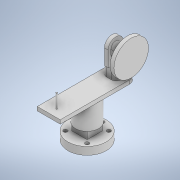
# Autodesk Inventor part: herramienta5
Saved by Autodesk Inventor 2022.3 (Build 263350000, 350)
## iProperties
Created: 2023-06-16
Part Number: herramienta5
Material: Generic
Document SubType Name: Modeling
Designer: crist
Density: 1 g/cm^3
Appearance: Default
Author: crist
Autodesk Inventor part; units mm, degrees
ref_plane "YZ Plane" through (0, 0, 0) normal (1, 0, 0) x (0, 1, 0)
ref_plane "XZ Plane" through (0, 0, 0) normal (0, 1, 0) x (-1, 0, 0)
ref_plane "XY Plane" through (0, 0, 0) normal (0, 0, 1) x (1, 0, 0)
sketch "Sketch1" plane through (0, 0, 0) normal (0, 1, 0) x (-1, 0, 0)
  line L0 (10, 10) -> (-10, 10)
  line L1 (-10, 10) -> (-10, -10)
  line L2 (-10, -10) -> (10, -10)
  line L3 (10, -10) -> (10, 10)
  line L4 (10, 10) -> (-10, -10) construction
  line L5 (-10, 10) -> (10, -10) construction
  point P0 (0, 0)
  dimension "d0" = 20
  dimension "d1" = 20
  constraints: 12 end point, 2 midpoint, 2 parallel, 1 horizontal, 1 perpendicular
  measures "d0" distance of L2.end L1.end
  measures "d1" distance of L1.end L0.end
extrude "Extrusion1" add sketch "Sketch1" along normal blind 20
sketch "Sketch2" plane through (0, 20, 0) normal (0, 1, 0) x (1, 0, 0)
  circle A0 centre (0, 0) radius 15
  dimension "d4" = 30
  constraints: 1 centre point, 1 coincident
  measures "d4" diameter of A0
extrude "Extrusion2" add sketch "Sketch2" along normal blind 30
sketch "Sketch3" plane through (0, 50, 0) normal (0, 1, 0) x (1, 0, 0)
  line L0 (-15, -50) -> (15, -50)
  line L1 (15, -50) -> (15, 50)
  line L2 (15, 50) -> (-15, 50)
  line L3 (-15, 50) -> (-15, -50)
  line L4 (-15, -50) -> (15, 50) construction
  line L5 (15, -50) -> (-15, 50) construction
  point P0 (0, 0)
  dimension "d7" = 30
  dimension "d8" = 100
  constraints: 12 end point, 2 midpoint, 2 parallel, 1 horizontal, 1 perpendicular
  measures "d7" distance of L2.end L1.end
  measures "d8" distance of L1.end L0.end
extrude "Extrusion3" add sketch "Sketch3" along normal blind 5
sketch "Sketch4" plane through (0, 55, 0) normal (0, 1, 0) x (1, 0, 0)
  arc A0 (-3, 41.5) -> (-3, 28.5) centre (-3, 35) ccw
  arc A1 (3, 28.5) -> (3, 41.5) centre (3, 35) ccw
  line L0 (-3, 28.5) -> (3, 28.5)
  line L1 (-3, 41.5) -> (3, 41.5)
  point P0 (0, 0)
  dimension "d11" = 13
  dimension "d12" = 13
  dimension "d13" = 3
  dimension "d14" = 3
  dimension "d15" = 35
  constraints: 4 end point, 4 point on circle, 2 centre point, 2 tangent, 1 horizontal
  measures "d11" diameter of A0
  measures "d12" diameter of A1
  measures "d13" horizontal distance of point (0, 0) A1.centre
  measures "d14" horizontal distance of point (0, 0) A0.centre
  measures "d15" vertical distance of point (0, 0) A0.centre
extrude "Extrusion4" cut sketch "Sketch4" against normal blind 5
fillet "Fillet1" radius 10 2 edges at (-15, 52.5, -50) (15, 52.5, -50)
sketch "Sketch5" plane through (0, 55, 0) normal (0, 1, 0) x (1, 0, 0)
  circle A0 centre (0, -39.6695) radius 1
  point P0 (0, 0)
  dimension "d19" = 2
  constraints: 1 centre point
  measures "d19" diameter of A0
extrude "Extrusion5" cut sketch "Sketch5" against normal blind 5
sketch "Sketch6" plane through (0, 0, 0) normal (0, -1, 0) x (1, 0, 0)
  circle A0 centre (-14.1421, 14.1421) radius 2.5
  circle A1 centre (-14.1421, -14.1421) radius 2.5
  line L0 (0, 0) -> (-14.1421, 14.1421)
  line L1 (0, 0) -> (0, -20)
  line L2 (0, 0) -> (-14.1421, -14.1421)
  circle A2 centre (0, -20) radius 2.5
  circle A3 centre (0, 0) radius 25
  line L3 (0, 0) -> (14.1421, 14.1421)
  circle A4 centre (14.1421, 14.1421) radius 2.5
  line L4 (0, 0) -> (14.1421, -14.1421)
  circle A5 centre (14.1421, -14.1421) radius 2.5
  line L5 (-10, 10) -> (10, 10)
  line L6 (10, 10) -> (10, -10)
  line L7 (10, -10) -> (-10, -10)
  line L8 (-10, -10) -> (-10, 10)
  line L9 (-10, 10) -> (10, -10) construction
  line L10 (10, 10) -> (-10, -10) construction
  dimension "d22" = 20
  dimension "d23" = 20
  dimension "d24" = 135
  dimension "d25" = 5
  dimension "d26" = 5
  dimension "d27" = 20
  dimension "d28" = 90
  dimension "d29" = 5
  dimension "d30" = 20
  dimension "d31" = 90
  dimension "d32" = 5
  dimension "d33" = 20
  dimension "d34" = 90
  dimension "d35" = 5
  dimension "d36" = 20
  dimension "d37" = 20
  constraints: 22 end point, 6 centre point, 6 coincident, 2 midpoint, 2 parallel, 1 horizontal, 1 perpendicular, 1 vertical
  measures "d22" distance of L2.start L1.end
  measures "d23" distance of L2.start L0.end
  measures "d24" angle of L0 L1
  measures "d25" diameter of A2
  measures "d26" diameter of A0
  measures "d27" distance of L2.start L3.end
  measures "d28" angle of L0 L3
  measures "d29" diameter of A4
  measures "d30" distance of L2.start L4.end
  measures "d31" angle of L3 L4
  measures "d32" diameter of A5
  measures "d33" distance of L2.start L2.end
  measures "d34" angle of L2 L4
  measures "d35" diameter of A1
  measures "d36" distance of L7.start L8.start
  measures "d37" distance of L5.end L7.start
extrude "Extrusion6" add sketch "Sketch6" against normal blind 10
sketch "Sketch7" plane through (0, 55, 0) normal (0, 1, 0) x (1, 0, 0)
  arc A0 (-3, 41.5) -> (-3, 28.5) centre (-3, 35) ccw
  arc A1 (3, 28.5) -> (3, 41.5) centre (3, 35) ccw
  line L0 (-3, 28.5) -> (3, 28.5)
  line L1 (-3, 41.5) -> (3, 41.5)
  point P0 (0, 0)
  dimension "d40" = 13
  dimension "d41" = 13
  constraints: 4 end point, 4 point on circle, 2 centre point, 2 tangent, 1 horizontal
  measures "d40" diameter of A0
  measures "d41" diameter of A1
extrude "Extrusion7" add sketch "Sketch7" along normal blind 15 and the other way blind 5
sketch "Sketch8" plane through (0, 70, 0) normal (0, 1, 0) x (1, 0, 0)
  line L0 (-2.5, 25) -> (2.5, 25)
  line L1 (2.5, 25) -> (2.5, 45)
  line L2 (2.5, 45) -> (-2.5, 45)
  line L3 (-2.5, 45) -> (-2.5, 25)
  line L4 (-2.5, 25) -> (2.5, 45) construction
  line L5 (2.5, 25) -> (-2.5, 45) construction
  arc A0 (-2.8422, 41.5) -> (-2.8422, 28.5) centre (-2.8422, 35) ccw construction
  arc A1 (3.1578, 28.5) -> (3.1578, 41.5) centre (3.1578, 35) ccw construction
  line L6 (-2.8422, 28.5) -> (3.1578, 28.5) construction
  line L7 (-2.8422, 41.5) -> (3.1578, 41.5) construction
  point P0 (0, 0)
  point P1 (0, 35)
  point P2 (0, 35)
  point P3 (0, 35)
  dimension "d46" = 5
  dimension "d47" = 20
  dimension "d48" = 13
  dimension "d49" = 13
  dimension "d50" = 35
  dimension "d51" = 0
  dimension "d52" = 0
  constraints: 16 end point, 4 midpoint, 4 point on circle, 2 centre point, 2 horizontal, 2 parallel, 2 tangent, 1 perpendicular
  measures "d46" distance of L2.end L1.end
  measures "d47" distance of L1.end L0.end
  measures "d48" diameter of A0
  measures "d49" diameter of A1
  measures "d50" vertical distance of point (0, 0) A0.centre
  measures "d51" vertical distance of A0.centre point (0, 35)
  measures "d52" horizontal distance of point (0, 0) point (0, 35)
extrude "Extrusion8" add sketch "Sketch8" along normal blind 30
sketch "Sketch9" plane through (2.5, 70, -25) normal (1, 0, 0) x (0, 0, -1)
  line L0 (0, 0) -> (0, 30) construction
  line L1 (16.5, 0) -> (20, 0) projected
  line L2 (0, 30) -> (20, 30) construction
  line L3 (20, 30) -> (20, 0) construction
  line L4 (20, 0) -> (0, 0) construction
  line L5 (0, 0) -> (0, 30) construction
  arc A0 (16.5, 19) -> (3.5, 19) centre (10, 19) ccw
  arc A1 (3.5, 13) -> (16.5, 13) centre (10, 13) ccw
  line L6 (3.5, 13) -> (3.5, 19)
  line L7 (16.5, 19) -> (16.5, 13)
  point P0 (-25, -70)
  point P1 (18.25, 0)
  dimension "d55" = 13
  dimension "d56" = 13
  dimension "d57" = 6
  dimension "d58" = 13
  constraints: 12 end point, 4 point on circle, 2 centre point, 2 parallel, 2 vertical, 1 horizontal, 1 midpoint, 1 perpendicular
  measures "d55" diameter of A0
  measures "d56" diameter of A1
  measures "d57" distance of L7.start L7.end
  measures "d58" vertical distance of point (18.25, 0) A1.centre
extrude "Extrusion9" cut sketch "Sketch9" against normal blind 30
fillet "Fillet2" radius 10 2 edges at (0, 100, -45) (0, 100, -25)
sketch "Sketch10" plane through (0, 50, 0) normal (0, -1, 0) x (1, 0, 0)
  circle A0 centre (0, 39.6695) radius 1 projected
  line L0 (0, 0) -> (0, 39.6695) construction
  circle A1 centre (0, 39.6695) radius 1
  constraints: 2 end point, 1 centre point, 1 coincident, 1 concentric, 1 vertical
extrude "Extrusion10" add sketch "Sketch10" against normal blind 23
sketch "Sketch11" plane through (2.5, 70, -25) normal (1, 0, 0) x (0, 0, -1)
  arc A0 (16.5, 19) -> (3.5, 19) centre (10, 19) ccw
  arc A1 (3.5, 13) -> (16.5, 13) centre (10, 13) ccw
  line L0 (3.5, 13) -> (3.5, 19)
  line L1 (16.5, 19) -> (16.5, 13)
  point P0 (-25, -70)
  dimension "d65" = 13
  dimension "d66" = 13
  dimension "d67" = 6
  constraints: 4 end point, 4 point on circle, 2 centre point, 2 vertical
  measures "d65" diameter of A0
  measures "d66" diameter of A1
  measures "d67" distance of L1.start L1.end
extrude "Extrusion11" add sketch "Sketch11" along normal blind 15 and the other way blind 5
sketch "Sketch13" plane through (17.5, 70, -25) normal (1, 0, 0) x (0, 0, -1)
  line L0 (3.5, 13) -> (3.5, 19) construction
  arc A0 (3.5, 13) -> (16.5, 13) centre (10, 13) ccw projected
  line L1 (3.5, 19) -> (16.5, 19) construction
  line L2 (16.5, 19) -> (16.5, 13) construction
  line L3 (16.5, 13) -> (3.5, 13) construction
  line L4 (3.5, 13) -> (3.5, 19) construction
  circle A1 centre (10, 16) radius 22.5
  point P0 (-25, -70)
  dimension "d76" = 45
  constraints: 8 end point, 2 parallel, 1 centre point, 1 horizontal, 1 perpendicular, 1 point on circle
  measures "d76" diameter of A1
extrude "Extrusion13" add sketch "Sketch13" along normal blind 5
body "Solid1"
